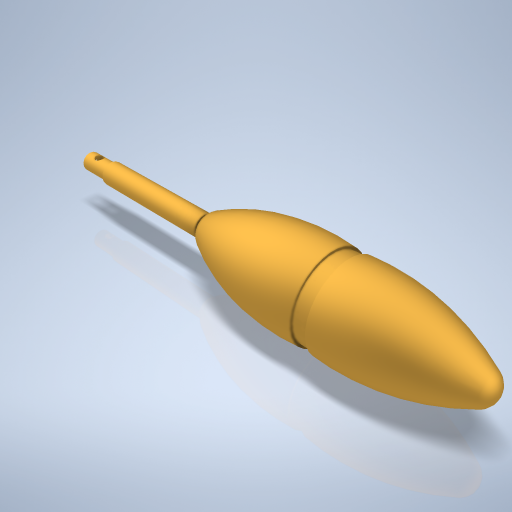
# Autodesk Inventor part: steuerkolben
Saved by Autodesk Inventor 2024.2 (Build 282272000, 272)
## iProperties
Created: 2024-04-07
Part Number: steuerkolben
Material: Messing, weicher Gelbton
Document SubType Name: Modeling
Designer: Fabri
Density: 8.47 g/cm^3
Appearance: Messing - satiniert
Author: Fabri
Autodesk Inventor part; units mm, degrees
ref_plane "YZ Plane" through (0, 0, 0) normal (1, 0, 0) x (0, 1, 0)
sketch "Skizze1" plane through (0, 0, 0) normal (0, 0, 1) x (1, 0, 0)
  line L0 (0, 0) -> (0, 2.1148)
  line L1 (0, 2.1148) -> (0.7513, 2.9749)
  arc A0 (29, 9) -> (1.8484, 3.855) centre (23.3975, -35.6499) ccw
  line L2 (29, 9) -> (29, 0)
  line L3 (29, 0) -> (0, 0)
  arc A1 (1.8484, 3.855) -> (0.7513, 2.9749) centre (3.7638, 0.3434) ccw
  point P0 (1.21, 3.5)
  dimension "d0" = 29
  dimension "d1" = 1.21
  dimension "d2" = 7
  dimension "d3" = 4
  dimension "d4" = 45
  dimension "d5" = 18
  dimension "d6" = 0.6868
  constraints: 8 end point, 5 point on circle, 2 centre point, 2 tangent, 2 vertical, 1 perpendicular, 1 point on line
  measures "d0" distance between parallel lines of L2 L0
  measures "d1" distance from line of point (1.21, 3.5) L0
  measures "d2" diameter of point (1.21, 3.5) L3
  measures "d3" radius of A1
  measures "d4" radius of A0
  measures "d5" diameter of L2.start L3
  measures "d6" diameter of A1.centre L3
revolve "Umdrehung1" add sketch "Skizze1" angle 360 about axis through (29, 0, 0) along (-1, 0, 0)
ref_plane "Arbeitsebene1" through (0, 0, 0) normal (0, 0, 1) x (1, 0, 0)
sketch "Skizze8" plane through (0, 0, 0) normal (0, 0, 1) x (1, 0, 0)
  line L0 (0.7513, 2.9749) -> (0, 2.1148) projected
  arc A0 (29, 9) -> (1.8484, 3.855) centre (23.3975, -35.6499) ccw projected
  arc A1 (1.8484, 3.855) -> (0.7513, 2.9749) centre (3.7638, 0.3434) ccw projected
  line L1 (0, 0) -> (39.6054, 0)
  line L2 (0, 2) -> (5.99, 2)
  line L3 (0, 2.1148) -> (0, -2.1148) projected
  line L4 (29, 9) -> (29, -9) projected
  arc A2 (29, 8.5) -> (13.2729, 7.6871) centre (23.3975, -35.6499) ccw
  arc A3 (13.2729, 7.6871) -> (5.99, 2) centre (15.7754, -3.0245) ccw
  point P0 (29, 0)
  dimension "d56" = 5.99
  dimension "d57" = 4
  dimension "d60" = 17
  dimension "d61" = 11
  constraints: 4 end point, 4 point on circle, 2 centre point, 2 horizontal, 2 point on line, 1 concentric, 1 tangent
  measures "d56" distance of L2.start L2.end
  measures "d57" diameter of L2 L1
  measures "d60" diameter of A2.start L1
  measures "d61" radius of A3
revolve "Umdrehung7" cut sketch "Skizze8" angle 360 about axis through (0, 0, 0) along (1, 0, 0) contours L2 A3 A2 L4 L1 L3
sketch "Skizze9" plane through (0, 0, 0) normal (0, 0, 1) x (1, 0, 0)
  line L0 (5.99, 2) -> (0, 2) projected
  line L1 (5.99, -2) -> (0, -2) projected
  line L2 (5.99, 2) -> (5.99, -2) projected
  line L3 (5.99, 2) -> (-0.01, 2)
  line L4 (-0.01, 2) -> (-0.01, 2.5)
  line L5 (-0.01, 2.5) -> (-27.01, 2.5)
  line L6 (-27.01, 2.5) -> (-27.01, 2)
  line L7 (-27.01, 2) -> (-34.01, 2)
  line L8 (-34.01, 2) -> (-34.01, 0)
  line L9 (-34.01, 0) -> (5.99, 0)
  line L10 (5.99, 2) -> (5.99, 0)
  point P0 (0, 0)
  dimension "d63" = 6
  dimension "d64" = 40
  dimension "d65" = 5
  dimension "d66" = 7
  constraints: 16 end point, 3 point on line, 2 perpendicular, 1 collinear, 1 midpoint, 1 parallel, 1 vertical
  measures "d63" distance of L0.start L3.end
  measures "d64" distance between parallel lines of L8 L2
  measures "d65" diameter of L5 L9
  measures "d66" distance between parallel lines of L6 L8
revolve "Umdrehung8" add sketch "Skizze9" angle 360 about axis through (-34.01, 0, 0) along (1, 0, 0)
sketch "Skizze10" plane through (-34.01, 0, 0) normal (-1, 0, 0) x (0, 0, 1)
  circle A0 centre (0, 0) radius 2 projected
  point P0 (0, 0)
  constraints: 1 coincident
hole "Bohrung1" at (-34.01, 0, 0) direction (1, 0, 0) diameter 2.5 depth 50
sketch "Skizze13" plane through (0, 0, 0) normal (0, 0, 1) x (1, 0, 0)
  arc A0 (29, 8.5) -> (13.2729, 7.6871) centre (23.3975, -35.6499) ccw projected
  arc A1 (29, 9) -> (1.8484, 3.855) centre (23.3975, -35.6499) ccw projected
  arc A2 (1.8484, -3.855) -> (29, -9) centre (23.3975, 35.6499) ccw projected
  arc A3 (13.2729, -7.6871) -> (29, -8.5) centre (23.3975, 35.6499) ccw projected
  line L0 (29, 8.5) -> (29, -8.5) projected
  line L1 (29, 8.5) -> (32, 8.5)
  line L2 (32, 8.5) -> (32, 9)
  arc A4 (57.7575, 3.0268) -> (32, 9) centre (35.1615, -35.8888) ccw
  arc A5 (59.5, 0) -> (57.7575, 3.0268) centre (56, 0) ccw
  line L3 (0, 0) -> (68.2278, 0)
  line L4 (29, 8.5) -> (29, 0)
  dimension "d92" = 3.5
  dimension "d93" = 18
  dimension "d94" = 17
  dimension "d95" = 30.5
  dimension "d96" = 45
  dimension "d97" = 3
  constraints: 8 end point, 4 point on circle, 3 point on line, 2 centre point, 2 horizontal, 1 midpoint, 1 perpendicular, 1 tangent
  measures "d92" radius of A5
  measures "d93" diameter of L2.end L3
  measures "d94" diameter of L1.end L3
  measures "d95" distance from line of A5.start L4
  measures "d96" radius of A4
  measures "d97" distance between parallel lines of L2 L4
revolve "Umdrehung10" add sketch "Skizze13" angle 360 about axis through (0, 0, 0) along (1, 0, 0)
sketch "Skizze15" plane through (0, 0, 0) normal (0, 0, 1) x (1, 0, 0)
  arc A0 (57.7575, 3.0268) -> (32, 9) centre (35.1615, -35.8888) ccw projected
  line L0 (29, 8.5) -> (32, 8.5) projected
  arc A1 (32, -9) -> (57.7575, -3.0268) centre (35.1615, 35.8888) ccw projected
  line L1 (29, -8.5) -> (32, -8.5) projected
  line L2 (13.2729, 7.6871) -> (13.2729, -7.6871) projected
  line L3 (29, 8.5) -> (29, -8.5) projected
  arc A2 (57.7575, -3.0268) -> (57.7575, 3.0268) centre (56, 0) ccw projected
  line L4 (29, 9) -> (29, -9) projected
  line L5 (29, 8) -> (32, 8)
  line L6 (0, 0) -> (69.0547, 0)
  line L7 (57.7575, -3.0268) -> (57.7575, 3.0268) projected
  arc A3 (57.7575, 1.8689) -> (32, 8) centre (35.1615, -35.8888) ccw
  arc A4 (58.5654, 0) -> (57.7575, 1.8689) centre (56, 0) ccw
  line L8 (29, 8) -> (29, 0)
  line L9 (29, 0) -> (58.5654, 0)
  point P0 (29, 0)
  point P1 (57.7575, 0)
  dimension "d99" = 16
  constraints: 8 end point, 4 point on circle, 4 point on line, 2 centre point, 2 concentric, 2 horizontal, 1 collinear, 1 midpoint, 1 vertical alignment
  measures "d99" diameter of L5 L6
revolve "Umdrehung11" cut sketch "Skizze15" angle 360 about axis through (0, 0, 0) along (1, 0, 0) contours L5 A3 L7 L6 L3
ref_plane "Arbeitsebene2" through (0, 0, 0) normal (0, 0, 1) x (1, 0, 0)
sketch "Skizze18" plane through (0, 0, 0) normal (0, 0, 1) x (1, 0, 0)
  circle A0 centre (-31.01, 0) radius 1
  line L0 (-34.01, -1.25) -> (-34.01, 1.25) projected
  point P0 (0, 0)
  dimension "d102" = 2
  dimension "d103" = 3
  constraints: 1 centre point, 1 horizontal alignment
  measures "d102" diameter of A0
  measures "d103" distance from line of L0 A0.centre
extrude "Extrusion1" cut sketch "Skizze18" along normal through all both and the other way through all
